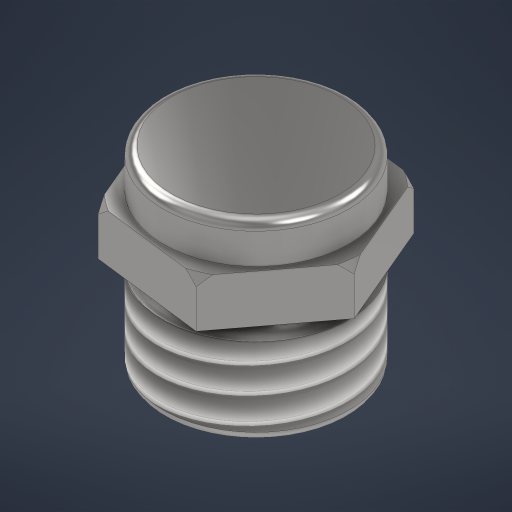
# Autodesk Inventor part: Pressure sensor
Saved by Autodesk Inventor 2023 (Build 270158000, 158)
## iProperties
Created: 2022-08-25
Part Number: Pressure sensor
Material: Stainless Steel
Document SubType Name: Modeling
Designer: Mike
Density: 8 g/cm^3
Appearance: Semi-Polished
Author: Mike
Autodesk Inventor part; units mm, degrees
ref_plane "YZ Plane" through (0, 0, 0) normal (1, 0, 0) x (0, 1, 0)
ref_plane "XZ Plane" through (0, 0, 0) normal (0, 1, 0) x (-1, 0, 0)
ref_plane "XY Plane" through (0, 0, 0) normal (0, 0, 1) x (1, 0, 0)
sketch "Sketch1" plane through (0, 0, 0) normal (0, 1, 0) x (-1, 0, 0)
  circle A0 centre (0, 0) radius 10.668
  dimension "d0" = 21.336
  constraints: 1 centre point, 1 coincident
  measures "d0" diameter of A0
extrude "Extrusion1" add sketch "Sketch1" along normal blind 10
sketch "Sketch2" plane through (0, 10, 0) normal (0, 1, 0) x (1, 0, 0)
  circle A0 centre (0, 0) radius 9.1
  dimension "d3" = 18.2
  constraints: 1 centre point, 1 coincident
  measures "d3" diameter of A0
extrude "Extrusion2" add sketch "Sketch2" along normal blind 2
fillet "Fillet1" radius 2 1 edges at (-9.1, 10, 0)
sketch "Sketch3" plane through (0, 12, 0) normal (0, 1, 0) x (1, 0, 0)
  circle A0 centre (0, 0) radius 12.95 construction
  line L0 (5.050414, -11.924589) -> (-7.80179, -10.336081)
  line L1 (-7.80179, -10.336081) -> (-12.852204, 1.588507)
  line L2 (-12.852204, 1.588507) -> (-5.050414, 11.924589)
  line L3 (-5.050414, 11.924589) -> (7.80179, 10.336081)
  line L4 (7.80179, 10.336081) -> (12.852204, -1.588507)
  line L5 (12.852204, -1.588507) -> (5.050414, -11.924589)
  dimension "d7" = 25.9
  dimension "d8" = 1.58851
  constraints: 12 end point, 2 coincident, 16 other
  measures "d8" vertical distance of L1.end point (0, 0)
extrude "Extrusion3" add sketch "Sketch3" along normal blind 5.5
ref_plane "Work Plane1" through (6.426098, 12, 0.794282) normal (-0.1226647, 0, 0.9924482) x (0.9924482, 0, 0.1226647)
sketch "Sketch4" plane through (6.426098, 12, 0.794282) normal (-0.1226647, 0, 0.9924482) x (0.9924482, 0, 0.1226647)
  line L0 (-12.95, 5.5) -> (-19.425, 5.5)
  line L1 (-18.793791, 5.5) -> (-20.475, 6.356619) construction
  line L2 (-20.475, 6.356619) -> (-20.475, 2.588061)
  line L3 (-20.475, 2.588061) -> (-18.793791, 5.5)
  line L4 (-19.425, 4.406714) -> (-19.425, 5.821617)
  line L5 (-19.425, 5.5) -> (-18.793791, 5.5)
  line L6 (-6.475, -15.671324) -> (-6.475, 10.027942)
  point P0 (-6.475, -12)
  dimension "d12" = 153
  dimension "d13" = 120
  dimension "d14" = 10
  dimension "d15" = 14
  dimension "d16" = 1.05
  constraints: 10 end point, 3 point on line, 1 collinear, 1 perpendicular, 1 vertical
  measures "d12" angle of L1 L0
  measures "d13" angle of L3 L0
  measures "d14" distance from line of point (-6.475, -12) L1
  measures "d15" distance from line of point (-6.475, -12) L2
  measures "d16" distance between parallel lines of L4 L2
revolve "Revolution1" cut sketch "Sketch4" angle 360 about axis through (-0.000004, -10, 0.000029) along (0, 1, 0)
sketch "Sketch5" plane through (0, 17.5, 0) normal (0, 1, 0) x (1, 0, 0)
  circle A0 centre (0, 0) radius 10.668
  dimension "d18" = 21.336
  constraints: 1 centre point, 1 coincident
  measures "d18" diameter of A0
extrude "Extrusion4" add sketch "Sketch5" along normal blind 4.5
fillet "Fillet2" radius 1 1 edges at (-10.668, 22, 0)
fillet "Fillet3" radius 1 1 edges at (10.668, 0, 0)
sketch "Sketch6" plane through (0, 0, 0) normal (0, -1, 0) x (1, 0, 0)
  circle A0 centre (0, 0) radius 1
  dimension "d23" = 2
  constraints: 1 centre point, 1 coincident
  measures "d23" diameter of A0
hole "Hole1" at (0, 0, 0) direction (0, 1, 0) diameter 2 depth 10 tip angle 118
thread "Thread1" size "M22x3" class "6g" standard "ANSI Metric M Profile" full length
body "Solid1"
